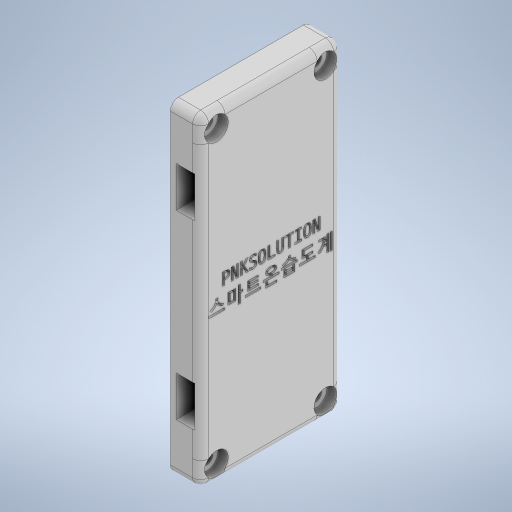
# Autodesk Inventor part: 222
Saved by Autodesk Inventor 2024 (Build 280153000, 153)
## iProperties
Created: 2025-04-29
Part Number: 222
Material: 일반
Document SubType Name: Modeling
Designer: User
Density: 1 g/cm^3
Appearance: 기본값
Author: User
Autodesk Inventor part; units mm, degrees
ref_plane "YZ Plane" through (0, 0, 0) normal (1, 0, 0) x (0, 1, 0)
ref_plane "XZ Plane" through (0, 0, 0) normal (0, 1, 0) x (-1, 0, 0)
ref_plane "XY Plane" through (0, 0, 0) normal (0, 0, 1) x (1, 0, 0)
sketch "스케치1" plane through (0, 0, 0) normal (1, 0, 0) x (0, 1, 0)
  line L0 (0, 0) -> (80, 0)
  line L1 (80, 0) -> (80, -35)
  line L2 (80, -35) -> (0, -35)
  line L3 (0, -35) -> (0, 0)
  dimension "d0" = 80
  dimension "d1" = 35
  constraints: 8 end point, 2 parallel, 1 horizontal, 1 perpendicular
  measures "d0" distance between parallel lines of L3 L1
  measures "d1" distance between parallel lines of L0 L2
extrude "돌출1" add sketch "스케치1" along normal blind 7.5
sketch "스케치2" plane through (7.5, 0, 0) normal (1, 0, 0) x (0, 0, -1)
  line L0 (35, 0) -> (35, 80) projected
  line L1 (35, 80) -> (27, 80)
  line L2 (27, 80) -> (27, 72)
  line L3 (27, 72) -> (35, 72)
  line L4 (35, 72) -> (35, 80)
  line L5 (35, 0) -> (27, 0)
  line L6 (27, 0) -> (27, 8)
  line L7 (27, 8) -> (35, 8)
  line L8 (35, 8) -> (35, 0)
  line L9 (0, 0) -> (8, 0)
  line L10 (8, 0) -> (8, 8)
  line L11 (8, 8) -> (0, 8)
  line L12 (0, 8) -> (0, 0)
  line L13 (0, 80) -> (8, 80)
  line L14 (8, 80) -> (8, 72)
  line L15 (8, 72) -> (0, 72)
  line L16 (0, 72) -> (0, 80)
  circle A0 centre (31, 76) radius 4
  circle A1 centre (4, 76) radius 4
  circle A2 centre (31, 4) radius 4
  circle A3 centre (4, 4) radius 4
  circle A4 centre (31, 4) radius 2.875
  circle A5 centre (4, 4) radius 2.875
  circle A6 centre (31, 76) radius 2.875
  circle A7 centre (4, 76) radius 2.875
  dimension "d4" = 8
  dimension "d5" = 5.75
  constraints: 32 end point, 12 tangent, 8 centre point, 8 parallel, 7 perpendicular, 6 point on line, 4 coincident, 4 horizontal, 3 equal radius
  measures "d4" distance of L6.end L7.end
  measures "d5" diameter of A6
extrude "돌출2" cut sketch "스케치2" against normal blind 2.5 contours A4 | A5 | A6 | A7
sketch "스케치3" plane through (5, 76, -31) normal (1, 0, 0) x (0, 0, -1)
  circle A0 centre (0, -72) radius 1.5
  circle A1 centre (-27, -72) radius 1.5
  circle A2 centre (0, 0) radius 1.5
  circle A3 centre (-27, 0) radius 1.5
  circle A4 centre (-27, 0) radius 2.875 projected
  circle A5 centre (0, 0) radius 2.875 projected
  circle A6 centre (0, -72) radius 2.875 projected
  circle A7 centre (-27, -72) radius 2.875 projected
  point P0 (-31, -76)
  dimension "d8" = 3
  constraints: 4 centre point, 4 concentric, 3 equal radius
  measures "d8" diameter of A2
extrude "돌출3" cut sketch "스케치3" against normal up to next contours A0 | A1 | A2 | A3
sketch "스케치4" plane through (0, 0, -35) normal (0, 0, -1) x (-1, 0, 0)
  line L0 (-7.5, 0) -> (-7.5, 80) projected
  line L1 (0, 80) -> (-7.5, 80) projected
  line L2 (0, 0) -> (0, 80) projected
  line L3 (0, 0) -> (-7.5, 0) projected
  line L4 (-6, 78.5) -> (-6, 1.5)
  line L5 (-6, 1.5) -> (-1.5, 1.5)
  line L6 (-1.5, 1.5) -> (-1.5, 78.5)
  line L7 (-1.5, 78.5) -> (-6, 78.5)
  line L8 (-6, 12.5) -> (-1.5, 12.5)
  line L9 (-1.5, 12.5) -> (-1.5, 22.5)
  line L10 (-1.5, 22.5) -> (-6, 22.5)
  line L11 (-6, 22.5) -> (-6, 12.5)
  line L12 (-6, 67.5) -> (-1.5, 67.5)
  line L13 (-1.5, 67.5) -> (-1.5, 57.5)
  line L14 (-1.5, 57.5) -> (-6, 57.5)
  line L15 (-6, 57.5) -> (-6, 67.5)
  point P0 (-6, 22.5)
  dimension "d14" = 1.5
  dimension "d15" = 12.5
  dimension "d16" = 12.5
  dimension "d17" = 10
  dimension "d18" = 10
  constraints: 24 end point, 4 parallel, 4 point on line, 2 horizontal, 2 perpendicular, 3 other
  measures "d14" distance between parallel lines of L0 L4
  measures "d15" distance between parallel lines of L3 L8
  measures "d16" distance between parallel lines of L12 L1
  measures "d17" distance between parallel lines of L10 L8
  measures "d18" distance between parallel lines of L14 L12
extrude "돌출4" cut sketch "스케치4" against normal up to next contours L12 L6 L14 L4 | L10 L6 L8 L4
fillet "모깎기1" radius 2 4 edges at (3.75, 80, -35) (3.75, 80, 0) (3.75, 0, -35) (3.75, 0, 0)
fillet "모깎기2" radius 1.9999 8 edges at (7.5, 79.4142, -0.5858) (7.5, 40, 0) (7.5, 0.5858, -0.5858) (7.5, 0, -17.5) (7.5, 0.5858, -34.4142) (7.5, 40, -35) (7.5, 79.4142, -34.4142) (7.5, 80, -17.5)
sketch "스케치5" plane through (7.5, 0, 0) normal (1, 0, 0) x (0, 0, -1)
  line L0 (1.9999, 78.0001) -> (33.0001, 78.0001) construction
  line L1 (33.0001, 78.0001) -> (33.0001, 1.9999) construction
  line L2 (33.0001, 1.9999) -> (1.9999, 1.9999) construction
  line L3 (1.9999, 1.9999) -> (1.9999, 78.0001) construction
  line L4 (28.9348, 1.9999) -> (6.0652, 1.9999) projected
  line L5 (33.0001, 73.9348) -> (33.0001, 6.0652) projected
  line L6 (1.9999, 6.0652) -> (1.9999, 73.9348) projected
  line L7 (6.0652, 78.0001) -> (28.9348, 78.0001) projected
  spline S0 degree 2 poles (7.2947, 43.4976) (7.2947, 43.0215) (6.7499, 42.5225) (6.1745, 42.5225) knots 0 0 0 1 2 2 2
  line L8 (6.1745, 42.5225) -> (5.9148, 42.5225)
  line L9 (5.9148, 42.5225) -> (5.9148, 41.3666)
  line L10 (5.9148, 41.3666) -> (5.4107, 41.3666)
  line L11 (5.4107, 41.3666) -> (5.4107, 44.4166)
  line L12 (5.4107, 44.4166) -> (6.1745, 44.4166)
  spline S1 degree 2 poles (6.1745, 44.4166) (6.4266, 44.4166) (6.839, 44.3097) (7.1318, 44.0882) (7.2947, 43.742) (7.2947, 43.4976) knots 0 0 0 1 2 3 4 4 4
  spline S2 degree 2 poles (6.7804, 43.4899) (6.7804, 43.6427) (6.6862, 43.8413) (6.5208, 43.9533) (6.2916, 43.9991) (6.1567, 43.9991) knots 0 0 0 1 2 3 4 4 4
  line L13 (6.1567, 43.9991) -> (5.9148, 43.9991)
  line L14 (5.9148, 43.9991) -> (5.9148, 42.9273)
  line L15 (5.9148, 42.9273) -> (6.0981, 42.9273)
  spline S3 degree 2 poles (6.0981, 42.9273) (6.2509, 42.9273) (6.508, 42.9757) (6.6837, 43.103) (6.7804, 43.3194) (6.7804, 43.4899) knots 0 0 0 1 2 3 4 4 4
  line L16 (8.7739, 41.3666) -> (8.1807, 43.3575)
  line L17 (8.1807, 43.3575) -> (8.0712, 43.9151)
  line L18 (8.0712, 43.9151) -> (8.0941, 43.3499)
  line L19 (8.0941, 43.3499) -> (8.0941, 41.3666)
  line L20 (8.0941, 41.3666) -> (7.6079, 41.3666)
  line L21 (7.6079, 41.3666) -> (7.6079, 44.4166)
  line L22 (7.6079, 44.4166) -> (8.2418, 44.4166)
  line L23 (8.2418, 44.4166) -> (8.8172, 42.4614)
  line L24 (8.8172, 42.4614) -> (8.9394, 41.8631)
  line L25 (8.9394, 41.8631) -> (8.9165, 42.4512)
  line L26 (8.9165, 42.4512) -> (8.9165, 44.4166)
  line L27 (8.9165, 44.4166) -> (9.4078, 44.4166)
  line L28 (9.4078, 44.4166) -> (9.4078, 41.3666)
  line L29 (9.4078, 41.3666) -> (8.7739, 41.3666)
  line L30 (10.8514, 43.0902) -> (11.8799, 41.3666)
  line L31 (11.8799, 41.3666) -> (11.2918, 41.3666)
  line L32 (11.2918, 41.3666) -> (10.5535, 42.716)
  line L33 (10.5535, 42.716) -> (10.3727, 42.4868)
  line L34 (10.3727, 42.4868) -> (10.3727, 41.3666)
  line L35 (10.3727, 41.3666) -> (9.8661, 41.3666)
  line L36 (9.8661, 41.3666) -> (9.8661, 44.4166)
  line L37 (9.8661, 44.4166) -> (10.3778, 44.4166)
  line L38 (10.3778, 44.4166) -> (10.3778, 43.215)
  line L39 (10.3778, 43.215) -> (11.2765, 44.4166)
  line L40 (11.2765, 44.4166) -> (11.8443, 44.4166)
  line L41 (11.8443, 44.4166) -> (10.8514, 43.0902)
  line L42 (12.0148, 42.054) -> (12.0861, 42.054)
  spline S4 degree 2 poles (12.0861, 42.054) (12.2974, 41.9064) (12.7353, 41.7536) (12.9237, 41.7536) knots 0 0 0 1 2 2 2
  spline S5 degree 2 poles (12.9237, 41.7536) (13.1783, 41.7536) (13.4533, 41.9573) (13.4533, 42.1941) knots 0 0 0 1 2 2 2
  spline S6 degree 2 poles (13.4533, 42.1941) (13.4533, 42.3621) (13.1885, 42.6371) (12.9899, 42.7262) knots 0 0 0 1 2 2 2
  spline S7 degree 2 poles (12.9899, 42.7262) (12.7608, 42.8331) (12.4196, 43.0368) (12.1956, 43.2557) (12.081, 43.5179) (12.081, 43.6834) knots 0 0 0 1 2 3 4 4 4
  spline S8 degree 2 poles (12.081, 43.6834) (12.081, 43.8845) (12.2363, 44.1824) (12.5011, 44.3759) (12.8473, 44.4701) (13.0408, 44.4701) knots 0 0 0 1 2 3 4 4 4
  spline S9 degree 2 poles (13.0408, 44.4701) (13.2369, 44.4701) (13.6569, 44.3886) (13.8352, 44.2588) knots 0 0 0 1 2 2 2
  line L43 (13.8352, 44.2588) -> (13.8352, 43.8234)
  line L44 (13.8352, 43.8234) -> (13.7588, 43.8234)
  spline S10 degree 2 poles (13.7588, 43.8234) (13.6009, 43.9278) (13.2191, 44.0348) (13.0485, 44.0348) knots 0 0 0 1 2 2 2
  spline S11 degree 2 poles (13.0485, 44.0348) (12.8321, 44.0348) (12.6029, 43.8769) (12.6029, 43.6962) knots 0 0 0 1 2 2 2
  spline S12 degree 2 poles (12.6029, 43.6962) (12.6029, 43.5307) (12.8244, 43.3295) (12.9848, 43.2608) knots 0 0 0 1 2 2 2
  spline S13 degree 2 poles (12.9848, 43.2608) (13.2649, 43.1437) (13.6519, 42.9146) (13.8886, 42.6676) (13.993, 42.3876) (13.993, 42.2221) knots 0 0 0 1 2 3 4 4 4
  spline S14 degree 2 poles (13.993, 42.2221) (13.993, 41.7536) (13.4227, 41.3081) (12.9135, 41.3081) knots 0 0 0 1 2 2 2
  spline S15 degree 2 poles (12.9135, 41.3081) (12.6539, 41.3081) (12.2032, 41.4557) (12.0148, 41.583) knots 0 0 0 1 2 2 2
  line L45 (12.0148, 41.583) -> (12.0148, 42.054)
  spline S16 degree 2 poles (15.2481, 44.465) (15.5307, 44.465) (15.9126, 44.2664) (16.1367, 43.8769) (16.2309, 43.2837) (16.2309, 42.8891) knots 0 0 0 1 2 3 4 4 4
  spline S17 degree 2 poles (16.2309, 42.8891) (16.2309, 42.4919) (16.1367, 41.8987) (15.9126, 41.5092) (15.5307, 41.3106) (15.2481, 41.3106) knots 0 0 0 1 2 3 4 4 4
  spline S18 degree 2 poles (15.2481, 41.3106) (14.963, 41.3106) (14.5862, 41.5092) (14.3622, 41.8987) (14.268, 42.4919) (14.268, 42.8891) knots 0 0 0 1 2 3 4 4 4
  spline S19 degree 2 poles (14.268, 42.8891) (14.268, 43.2837) (14.3622, 43.8769) (14.5862, 44.2664) (14.963, 44.465) (15.2481, 44.465) knots 0 0 0 1 2 3 4 4 4
  spline S20 degree 2 poles (15.2481, 44.0526) (14.9834, 44.0526) (14.7619, 43.495) (14.7619, 42.8891) knots 0 0 0 1 2 2 2
  spline S21 degree 2 poles (14.7619, 42.8891) (14.7619, 42.2806) (14.9834, 41.7231) (15.2481, 41.7231) knots 0 0 0 1 2 2 2
  spline S22 degree 2 poles (15.2481, 41.7231) (15.5078, 41.7231) (15.7471, 42.2806) (15.7471, 42.8891) knots 0 0 0 1 2 2 2
  spline S23 degree 2 poles (15.7471, 42.8891) (15.7471, 43.495) (15.5078, 44.0526) (15.2481, 44.0526) knots 0 0 0 1 2 2 2
  line L46 (18.4789, 41.7893) -> (18.4789, 41.3666)
  line L47 (18.4789, 41.3666) -> (16.6866, 41.3666)
  line L48 (16.6866, 41.3666) -> (16.6866, 44.4166)
  line L49 (16.6866, 44.4166) -> (17.1907, 44.4166)
  line L50 (17.1907, 44.4166) -> (17.1907, 41.7893)
  line L51 (17.1907, 41.7893) -> (18.4789, 41.7893)
  spline S24 degree 2 poles (19.7493, 41.3106) (19.3114, 41.3106) (18.8582, 41.8402) (18.8582, 42.3315) knots 0 0 0 1 2 2 2
  line L52 (18.8582, 42.3315) -> (18.8582, 44.4166)
  line L53 (18.8582, 44.4166) -> (19.3623, 44.4166)
  line L54 (19.3623, 44.4166) -> (19.3623, 42.3723)
  spline S25 degree 2 poles (19.3623, 42.3723) (19.3623, 42.2373) (19.398, 41.998) (19.4871, 41.8275) (19.6347, 41.7282) (19.7493, 41.7282) knots 0 0 0 1 2 3 4 4 4
  spline S26 degree 2 poles (19.7493, 41.7282) (19.8613, 41.7282) (20.0141, 41.8275) (20.0981, 41.998) (20.1337, 42.2373) (20.1337, 42.3723) knots 0 0 0 1 2 3 4 4 4
  line L55 (20.1337, 42.3723) -> (20.1337, 44.4166)
  line L56 (20.1337, 44.4166) -> (20.6378, 44.4166)
  line L57 (20.6378, 44.4166) -> (20.6378, 42.3315)
  spline S27 degree 2 poles (20.6378, 42.3315) (20.6378, 41.8402) (20.1847, 41.3106) (19.7493, 41.3106) knots 0 0 0 1 2 2 2
  line L58 (22.2468, 41.3666) -> (21.7453, 41.3666)
  line L59 (21.7453, 41.3666) -> (21.7453, 43.994)
  line L60 (21.7453, 43.994) -> (20.9383, 43.994)
  line L61 (20.9383, 43.994) -> (20.9383, 44.4166)
  line L62 (20.9383, 44.4166) -> (23.0539, 44.4166)
  line L63 (23.0539, 44.4166) -> (23.0539, 43.994)
  line L64 (23.0539, 43.994) -> (22.2468, 43.994)
  line L65 (22.2468, 43.994) -> (22.2468, 41.3666)
  line L66 (25.0219, 44.4166) -> (25.0219, 43.994)
  line L67 (25.0219, 43.994) -> (24.4949, 43.994)
  line L68 (24.4949, 43.994) -> (24.4949, 41.7867)
  line L69 (24.4949, 41.7867) -> (25.1085, 41.7867)
  line L70 (25.1085, 41.7867) -> (25.1085, 41.3641)
  line L71 (25.1085, 41.3641) -> (23.3772, 41.3641)
  line L72 (23.3772, 41.3641) -> (23.3772, 41.7867)
  line L73 (23.3772, 41.7867) -> (23.9933, 41.7867)
  line L74 (23.9933, 41.7867) -> (23.9933, 43.994)
  line L75 (23.9933, 43.994) -> (23.4663, 43.994)
  line L76 (23.4663, 43.994) -> (23.4663, 44.4166)
  line L77 (23.4663, 44.4166) -> (25.0219, 44.4166)
  spline S28 degree 2 poles (26.4883, 44.465) (26.7709, 44.465) (27.1528, 44.2664) (27.3769, 43.8769) (27.4711, 43.2837) (27.4711, 42.8891) knots 0 0 0 1 2 3 4 4 4
  spline S29 degree 2 poles (27.4711, 42.8891) (27.4711, 42.4919) (27.3769, 41.8987) (27.1528, 41.5092) (26.7709, 41.3106) (26.4883, 41.3106) knots 0 0 0 1 2 3 4 4 4
  spline S30 degree 2 poles (26.4883, 41.3106) (26.2032, 41.3106) (25.8264, 41.5092) (25.6024, 41.8987) (25.5082, 42.4919) (25.5082, 42.8891) knots 0 0 0 1 2 3 4 4 4
  spline S31 degree 2 poles (25.5082, 42.8891) (25.5082, 43.2837) (25.6024, 43.8769) (25.8264, 44.2664) (26.2032, 44.465) (26.4883, 44.465) knots 0 0 0 1 2 3 4 4 4
  spline S32 degree 2 poles (26.4883, 44.0526) (26.2236, 44.0526) (26.0021, 43.495) (26.0021, 42.8891) knots 0 0 0 1 2 2 2
  spline S33 degree 2 poles (26.0021, 42.8891) (26.0021, 42.2806) (26.2236, 41.7231) (26.4883, 41.7231) knots 0 0 0 1 2 2 2
  spline S34 degree 2 poles (26.4883, 41.7231) (26.748, 41.7231) (26.9873, 42.2806) (26.9873, 42.8891) knots 0 0 0 1 2 2 2
  spline S35 degree 2 poles (26.9873, 42.8891) (26.9873, 43.495) (26.748, 44.0526) (26.4883, 44.0526) knots 0 0 0 1 2 2 2
  line L78 (29.0062, 41.3666) -> (28.413, 43.3575)
  line L79 (28.413, 43.3575) -> (28.3036, 43.9151)
  line L80 (28.3036, 43.9151) -> (28.3265, 43.3499)
  line L81 (28.3265, 43.3499) -> (28.3265, 41.3666)
  line L82 (28.3265, 41.3666) -> (27.8402, 41.3666)
  line L83 (27.8402, 41.3666) -> (27.8402, 44.4166)
  line L84 (27.8402, 44.4166) -> (28.4741, 44.4166)
  line L85 (28.4741, 44.4166) -> (29.0495, 42.4614)
  line L86 (29.0495, 42.4614) -> (29.1717, 41.8631)
  line L87 (29.1717, 41.8631) -> (29.1488, 42.4512)
  line L88 (29.1488, 42.4512) -> (29.1488, 44.4166)
  line L89 (29.1488, 44.4166) -> (29.6402, 44.4166)
  line L90 (29.6402, 44.4166) -> (29.6402, 41.3666)
  line L91 (29.6402, 41.3666) -> (29.0062, 41.3666)
  spline S36 degree 2 poles (4.2638, 38.8625) (4.5108, 38.4093) (5.2389, 37.8059) (5.7735, 37.6074) knots 0 0 0 1 2 2 2
  line L92 (5.7735, 37.6074) -> (5.4375, 37.1847)
  spline S37 degree 2 poles (5.4375, 37.1847) (4.9741, 37.3528) (4.2816, 37.9129) (4.0347, 38.3049) knots 0 0 0 1 2 2 2
  spline S38 degree 2 poles (4.0347, 38.3049) (3.8055, 37.9103) (3.0647, 37.3375) (2.6268, 37.1822) knots 0 0 0 1 2 2 2
  line L93 (2.6268, 37.1822) -> (2.2856, 37.6048)
  spline S39 degree 2 poles (2.2856, 37.6048) (2.6446, 37.7347) (3.2073, 38.0656) (3.5841, 38.5213) (3.775, 39.1145) (3.7648, 39.5066) knots 0 0 0 1 2 3 4 4 4
  line L94 (3.7648, 39.5066) -> (4.3224, 39.5066)
  spline S40 degree 2 poles (4.3224, 39.5066) (4.3326, 39.3335) (4.2995, 39.0152) (4.2638, 38.8625) knots 0 0 0 1 2 2 2
  line L95 (5.9365, 36.5788) -> (5.9365, 36.1155)
  line L96 (5.9365, 36.1155) -> (2.0794, 36.1155)
  line L97 (2.0794, 36.1155) -> (2.0794, 36.5788)
  line L98 (2.0794, 36.5788) -> (5.9365, 36.5788)
  line L99 (8.709, 36.6348) -> (6.7995, 36.6348)
  line L100 (6.7995, 36.6348) -> (6.7995, 39.3513)
  line L101 (6.7995, 39.3513) -> (8.709, 39.3513)
  line L102 (8.709, 39.3513) -> (8.709, 36.6348)
  line L103 (10.5166, 37.7958) -> (9.8648, 37.7958)
  line L104 (9.8648, 37.7958) -> (9.8648, 35.5299)
  line L105 (9.8648, 35.5299) -> (9.3073, 35.5299)
  line L106 (9.3073, 35.5299) -> (9.3073, 39.6975)
  line L107 (9.3073, 39.6975) -> (9.8648, 39.6975)
  line L108 (9.8648, 39.6975) -> (9.8648, 38.2718)
  line L109 (9.8648, 38.2718) -> (10.5166, 38.2718)
  line L110 (10.5166, 38.2718) -> (10.5166, 37.7958)
  line L111 (8.1565, 37.0982) -> (8.1565, 38.893)
  line L112 (8.1565, 38.893) -> (7.3622, 38.893)
  line L113 (7.3622, 38.893) -> (7.3622, 37.0982)
  line L114 (7.3622, 37.0982) -> (8.1565, 37.0982)
  line L115 (11.6826, 37.1211) -> (11.6826, 39.3869)
  line L116 (11.6826, 39.3869) -> (14.3303, 39.3869)
  line L117 (14.3303, 39.3869) -> (14.3303, 38.9185)
  line L118 (14.3303, 38.9185) -> (12.23, 38.9185)
  line L119 (12.23, 38.9185) -> (12.23, 38.5061)
  line L120 (12.23, 38.5061) -> (14.2565, 38.5061)
  line L121 (14.2565, 38.5061) -> (14.2565, 38.0554)
  line L122 (14.2565, 38.0554) -> (12.23, 38.0554)
  line L123 (12.23, 38.0554) -> (12.23, 37.5794)
  line L124 (12.23, 37.5794) -> (14.3838, 37.5794)
  line L125 (14.3838, 37.5794) -> (14.3838, 37.1211)
  line L126 (14.3838, 37.1211) -> (11.6826, 37.1211)
  line L127 (14.9286, 36.5737) -> (14.9286, 36.1104)
  line L128 (14.9286, 36.1104) -> (11.0716, 36.1104)
  line L129 (11.0716, 36.1104) -> (11.0716, 36.5737)
  line L130 (11.0716, 36.5737) -> (14.9286, 36.5737)
  spline S41 degree 2 poles (18.885, 38.809) (18.885, 38.4577) (18.3147, 37.9714) (17.7699, 37.923) knots 0 0 0 1 2 2 2
  line L131 (17.7699, 37.923) -> (17.7699, 37.5539)
  line L132 (17.7699, 37.5539) -> (19.4705, 37.5539)
  line L133 (19.4705, 37.5539) -> (19.4705, 37.0854)
  line L134 (19.4705, 37.0854) -> (15.5295, 37.0854)
  line L135 (15.5295, 37.0854) -> (15.5295, 37.5539)
  line L136 (15.5295, 37.5539) -> (17.2072, 37.5539)
  line L137 (17.2072, 37.5539) -> (17.2072, 37.923)
  spline S42 degree 2 poles (17.2072, 37.923) (16.6726, 37.9816) (16.1099, 38.4577) (16.1099, 38.809) knots 0 0 0 1 2 2 2
  spline S43 degree 2 poles (16.1099, 38.809) (16.1099, 39.0025) (16.2958, 39.3309) (16.6446, 39.5728) (17.1614, 39.7128) (17.5, 39.7128) knots 0 0 0 1 2 3 4 4 4
  spline S44 degree 2 poles (17.5, 39.7128) (17.8335, 39.7128) (18.3503, 39.5728) (18.7017, 39.3309) (18.885, 39.0025) (18.885, 38.809) knots 0 0 0 1 2 3 4 4 4
  line L138 (18.9333, 35.5935) -> (16.143, 35.5935)
  line L139 (16.143, 35.5935) -> (16.143, 36.8156)
  line L140 (16.143, 36.8156) -> (16.6904, 36.8156)
  line L141 (16.6904, 36.8156) -> (16.6904, 36.0645)
  line L142 (16.6904, 36.0645) -> (18.9333, 36.0645)
  line L143 (18.9333, 36.0645) -> (18.9333, 35.5935)
  spline S45 degree 2 poles (18.2969, 38.7988) (18.2969, 38.893) (18.2052, 39.0611) (18.0168, 39.1909) (17.7164, 39.2622) (17.5, 39.2622) knots 0 0 0 1 2 3 4 4 4
  spline S46 degree 2 poles (17.5, 39.2622) (17.2785, 39.2622) (16.973, 39.1909) (16.7795, 39.0611) (16.6955, 38.893) (16.6955, 38.7988) knots 0 0 0 1 2 3 4 4 4
  spline S47 degree 2 poles (16.6955, 38.7988) (16.6955, 38.7046) (16.7795, 38.5468) (16.9704, 38.4297) (17.276, 38.3635) (17.4949, 38.3635) knots 0 0 0 1 2 3 4 4 4
  spline S48 degree 2 poles (17.4949, 38.3635) (17.7113, 38.3635) (18.0168, 38.4297) (18.2103, 38.5468) (18.2969, 38.7046) (18.2969, 38.7988) knots 0 0 0 1 2 3 4 4 4
  line L144 (20.6569, 35.5935) -> (20.6569, 37.2382)
  line L145 (20.6569, 37.2382) -> (21.2043, 37.2382)
  line L146 (21.2043, 37.2382) -> (21.2043, 36.892)
  line L147 (21.2043, 36.892) -> (22.8235, 36.892)
  line L148 (22.8235, 36.892) -> (22.8235, 37.2382)
  line L149 (22.8235, 37.2382) -> (23.3709, 37.2382)
  line L150 (23.3709, 37.2382) -> (23.3709, 35.5935)
  line L151 (23.3709, 35.5935) -> (20.6569, 35.5935)
  spline S49 degree 2 poles (22.2507, 39.2113) (22.4798, 38.9516) (23.2588, 38.6003) (23.7069, 38.5392) knots 0 0 0 1 2 2 2
  line L152 (23.7069, 38.5392) -> (23.4345, 38.1064)
  spline S50 degree 2 poles (23.4345, 38.1064) (22.9839, 38.1827) (22.2507, 38.5646) (21.9732, 38.8167) knots 0 0 0 1 2 2 2
  spline S51 degree 2 poles (21.9732, 38.8167) (21.8382, 38.6766) (21.5022, 38.4348) (21.1279, 38.2464) (20.7359, 38.1114) (20.5424, 38.0783) knots 0 0 0 1 2 3 4 4 4
  line L153 (20.5424, 38.0783) -> (20.2776, 38.501)
  spline S52 degree 2 poles (20.2776, 38.501) (20.6187, 38.5595) (21.1763, 38.7861) (21.5684, 39.0942) (21.7797, 39.4811) (21.7797, 39.6975) knots 0 0 0 1 2 3 4 4 4
  line L154 (21.7797, 39.6975) -> (22.35, 39.6975)
  spline S53 degree 2 poles (22.35, 39.6975) (22.3627, 39.4531) (22.2507, 39.2113) knots 0 0 0 1 1 1
  line L155 (23.9666, 37.9256) -> (23.9666, 37.4622)
  line L156 (23.9666, 37.4622) -> (20.0255, 37.4622)
  line L157 (20.0255, 37.4622) -> (20.0255, 37.9256)
  line L158 (20.0255, 37.9256) -> (23.9666, 37.9256)
  line L159 (22.826, 36.4642) -> (21.2018, 36.4642)
  line L160 (21.2018, 36.4642) -> (21.2018, 36.0467)
  line L161 (21.2018, 36.0467) -> (22.826, 36.0467)
  line L162 (22.826, 36.0467) -> (22.826, 36.4642)
  line L163 (25.1428, 37.3324) -> (25.1428, 39.3589)
  line L164 (25.1428, 39.3589) -> (27.8364, 39.3589)
  line L165 (27.8364, 39.3589) -> (27.8364, 38.8829)
  line L166 (27.8364, 38.8829) -> (25.7055, 38.8829)
  line L167 (25.7055, 38.8829) -> (25.7055, 37.8034)
  line L168 (25.7055, 37.8034) -> (27.8746, 37.8034)
  line L169 (27.8746, 37.8034) -> (27.8746, 37.3324)
  line L170 (27.8746, 37.3324) -> (26.8002, 37.3324)
  line L171 (26.8002, 37.3324) -> (26.8002, 36.5788)
  line L172 (26.8002, 36.5788) -> (28.4423, 36.5788)
  line L173 (28.4423, 36.5788) -> (28.4423, 36.1155)
  line L174 (28.4423, 36.1155) -> (24.5369, 36.1155)
  line L175 (24.5369, 36.1155) -> (24.5369, 36.5788)
  line L176 (24.5369, 36.5788) -> (26.2325, 36.5788)
  line L177 (26.2325, 36.5788) -> (26.2325, 37.3324)
  line L178 (26.2325, 37.3324) -> (25.1428, 37.3324)
  line L179 (30.9068, 38.6588) -> (31.3116, 38.6588)
  line L180 (31.3116, 38.6588) -> (31.3116, 39.6517)
  line L181 (31.3116, 39.6517) -> (31.8284, 39.6517)
  line L182 (31.8284, 39.6517) -> (31.8284, 35.6343)
  line L183 (31.8284, 35.6343) -> (31.3116, 35.6343)
  line L184 (31.3116, 35.6343) -> (31.3116, 37.2611)
  line L185 (31.3116, 37.2611) -> (30.754, 37.2611)
  line L186 (30.754, 37.2611) -> (30.754, 37.7245)
  line L187 (30.754, 37.7245) -> (31.3167, 37.7245)
  line L188 (31.3167, 37.7245) -> (31.3167, 38.1955)
  line L189 (31.3167, 38.1955) -> (30.8075, 38.1955)
  spline S54 degree 2 poles (30.8075, 38.1955) (30.6547, 37.6379) (30.0259, 36.7341) (29.4963, 36.3828) knots 0 0 0 1 2 2 2
  line L190 (29.4963, 36.3828) -> (29.1043, 36.7392)
  spline S55 degree 2 poles (29.1043, 36.7392) (29.4505, 36.9607) (29.9215, 37.4673) (30.2194, 38.0122) (30.3619, 38.5952) (30.3772, 38.893) knots 0 0 0 1 2 3 4 4 4
  spline S56 degree 2 poles (30.3772, 38.893) (30.1965, 38.8829) (29.8909, 38.8829) (29.7153, 38.8829) knots 0 0 0 1 2 2 2
  line L191 (29.7153, 38.8829) -> (29.3334, 38.8829)
  line L192 (29.3334, 38.8829) -> (29.3334, 39.3411)
  line L193 (29.3334, 39.3411) -> (29.9622, 39.3411)
  spline S57 degree 2 poles (29.9622, 39.3411) (30.2321, 39.3411) (30.7362, 39.3462) (30.9704, 39.3513) knots 0 0 0 1 2 2 2
  spline S58 degree 2 poles (30.9704, 39.3513) (30.9602, 39.1705) (30.9348, 38.8243) (30.9068, 38.6588) knots 0 0 0 1 2 2 2
  line L194 (32.6558, 35.5299) -> (32.1339, 35.5299)
  line L195 (32.1339, 35.5299) -> (32.1339, 39.6975)
  line L196 (32.1339, 39.6975) -> (32.6558, 39.6975)
  line L197 (32.6558, 39.6975) -> (32.6558, 35.5299)
  point P0 (0, 0)
  dimension "d11" = 2
  constraints: 4 collinear, 2 other
extrude "돌출5" cut sketch "스케치5" against normal blind 1
